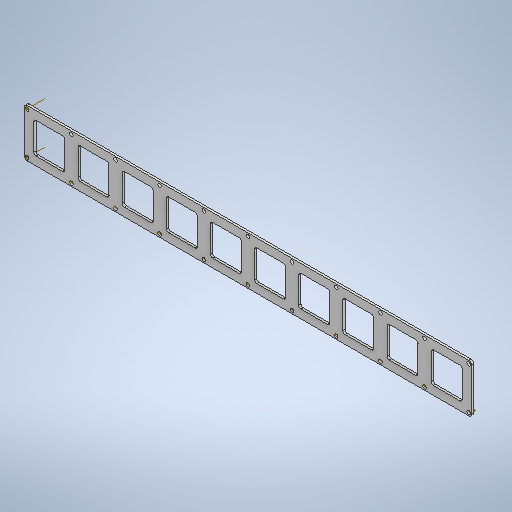
# Autodesk Inventor part: Maske
Saved by Autodesk Inventor 2025.2 (Build 292293000, 293)
## iProperties
Created: 2025-01-20
Part Number: Maske
Material: Generisch
Document SubType Name: Modeling
Designer: gorenfl4
Density: 1 g/cm^3
Appearance: Vorgabe
Author: gorenfl4
Autodesk Inventor part; units mm, degrees
ref_plane "YZ Plane" through (0, 0, 0) normal (1, 0, 0) x (0, 1, 0)
ref_plane "XZ Plane" through (0, 0, 0) normal (0, 1, 0) x (-1, 0, 0)
ref_plane "XY Plane" through (0, 0, 0) normal (0, 0, 1) x (1, 0, 0)
sketch "Skizze1" plane through (0, 0, 0) normal (0, 1, 0) x (-1, 0, 0)
  arc A0 (-143, 18) -> (-145, 16) centre (-143, 16) ccw
  line L0 (-145, 16) -> (-145, -12.6)
  line L1 (-143, 18) -> (157, 18)
  line L2 (-143, -14.6) -> (157, -14.6)
  line L3 (159, 16.0803) -> (159, -12.6)
  arc A1 (157, -14.6) -> (159, -12.6) centre (157, -12.6) ccw
  arc A2 (159, 16) -> (157, 18) centre (157, 16) ccw
  line L4 (157, 16) -> (157, 18) construction
  line L5 (157, 16) -> (159, 16) construction
  arc A3 (-145, -12.6) -> (-143, -14.6) centre (-143, -12.6) ccw
  point P0 (0, 0)
  dimension "d0" = 90
  dimension "d1" = 32.6
  dimension "d2" = 304
  dimension "d3" = 2
  dimension "d4" = 2
  dimension "d5" = 2
  dimension "d6" = 2
  dimension "d7" = 18
  dimension "d8" = 145
  constraints: 12 end point, 8 point on circle, 8 tangent, 4 centre point, 1 perpendicular, 1 vertical
  measures "d0" angle of L5 L4
  measures "d1" distance between parallel lines of L1 L2
  measures "d2" distance between parallel lines of L0 L3
  measures "d3" radius of A2
  measures "d4" radius of A1
  measures "d5" radius of A0
  measures "d6" radius of A3
  measures "d7" distance from line of point (0, 0) L1
  measures "d8" distance from line of point (0, 0) L0
extrude "Extrusion1" add sketch "Skizze1" along normal blind 1.5
sketch "Skizze2" plane through (0, 1.5, 0) normal (0, 1, 0) x (1, 0, 0)
  line L0 (-152.5, 8.8) -> (-131.5, 8.8)
  line L1 (-131.5, 8.8) -> (-131.5, -12.2)
  line L2 (-131.5, -12.2) -> (-152.5, -12.2)
  line L3 (-152.5, -12.2) -> (-152.5, 8.8)
  line L4 (-159, 12.6) -> (-159, -16) projected
  line L5 (143, 14.6) -> (-157, 14.6) projected
  point P0 (0, 0)
  dimension "d11" = 21
  dimension "d12" = 21
  dimension "d13" = 6.5
  dimension "d14" = 5.8
  constraints: 8 end point, 2 parallel, 1 horizontal, 1 perpendicular
  measures "d11" distance of L0.end L1.end
  measures "d12" distance of L0.start L0.end
  measures "d13" distance between parallel lines of L4 L3
  measures "d14" distance between parallel lines of L5 L0
extrude "Extrusion2" cut sketch "Skizze2" against normal through all
pattern_linear "Rechteckige Anordnung1" count 10 spacing 30 along (1, 0, 0) of "Extrusion2"
hole "Bohrung1" at (-157, 1.5, -12.6) direction (0, -1, 0) diameter 2.4 depth 4.2 tip angle 118
pattern_of_nothing "Rechteckige Anordnung2"
pattern_linear "Rechteckige Anordnung3" count 11 spacing 30 along (1, 0, 0) of "Bohrung1"
hole "Bohrung2" at (-157, 1.5, 16) direction (0, -1, 0) diameter 2.4 depth 4.2 tip angle 118
pattern_linear "Rechteckige Anordnung4" count 11 spacing 30 along (1, 0, 0) of "Bohrung2"
fillet "Rundung1" radius 1.5 4 edges at (-152.5, 0.75, -8.8) (-152.5, 0.75, 12.2) (-131.5, 0.75, -8.8) (-131.5, 0.75, 12.2)
fillet "Rundung2" radius 1.5 36 edges at (-101.5, 0.75, 12.2) (-71.5, 0.75, 12.2) (-41.5, 0.75, 12.2) (-11.5, 0.75, 12.2) (18.5, 0.75, 12.2) (48.5, 0.75, 12.2) (78.5, 0.75, 12.2) (108.5, 0.75, 12.2) (138.5, 0.75, 12.2) (-101.5, 0.75, -8.8) (-71.5, 0.75, -8.8) (-41.5, 0.75, -8.8) (-11.5, 0.75, -8.8) (18.5, 0.75, -8.8) (48.5, 0.75, -8.8) (78.5, 0.75, -8.8) (108.5, 0.75, -8.8) (138.5, 0.75, -8.8) (-122.5, 0.75, -8.8) (-92.5, 0.75, -8.8) (-62.5, 0.75, -8.8) (-32.5, 0.75, -8.8) (-2.5, 0.75, -8.8) (27.5, 0.75, -8.8) (57.5, 0.75, -8.8) (87.5, 0.75, -8.8) (117.5, 0.75, -8.8) (-122.5, 0.75, 12.2) (-92.5, 0.75, 12.2) (-62.5, 0.75, 12.2) (-32.5, 0.75, 12.2) (-2.5, 0.75, 12.2) (27.5, 0.75, 12.2) (57.5, 0.75, 12.2) (87.5, 0.75, 12.2) (117.5, 0.75, 12.2)
